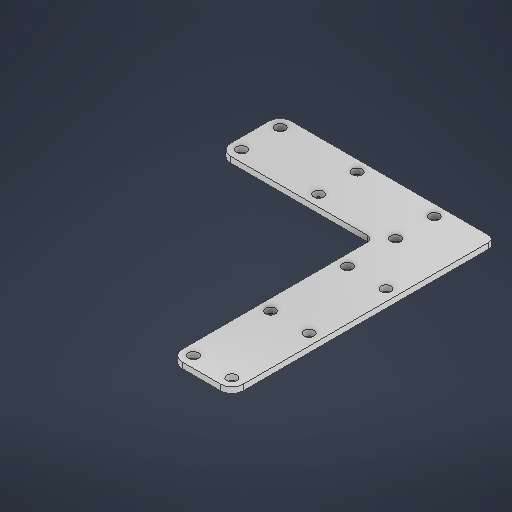
# Autodesk Inventor part: CNC-003-StructureGusset3
Saved by Autodesk Inventor 2026.2 (Build 302298000, 298)
## iProperties
Created: 2026-06-14
Part Number: CNC-003-StructureGusset3
Material: Steel AISI 1080
Document SubType Name: Modeling
Designer: Kenji
Density: 7.85 g/cm^3
Appearance: Aluminum - Dark
Author: Kenji
Autodesk Inventor part; units mm, degrees
ref_plane "YZ Plane" through (0, 0, 0) normal (1, 0, 0) x (0, 1, 0)
ref_plane "XZ Plane" through (0, 0, 0) normal (0, 1, 0) x (-1, 0, 0)
ref_plane "XY Plane" through (0, 0, 0) normal (0, 0, 1) x (1, 0, 0)
sketch "Sketch1" plane through (0, 0, 0) normal (0, 1, 0) x (-1, 0, 0)
  circle A0 centre (0, 0) radius 2.6
  line L0 (0, 0) -> (0, -2.6) construction
  line L1 (0, 0) -> (-2.6, 0) construction
  circle A1 centre (-20, 0) radius 2.6
  circle A2 centre (0, 40) radius 2.6
  circle A3 centre (-20, 40) radius 2.6
  circle A4 centre (0, 80) radius 2.6
  circle A5 centre (-20, 80) radius 2.6
  circle A6 centre (0, -25) radius 2.6
  line L2 (0, -25) -> (2.6, -25) construction
  line L3 (0, -25) -> (0, -27.6) construction
  circle A7 centre (40, -25) radius 2.6
  circle A8 centre (80, -25) radius 2.6
  circle A9 centre (0, -45) radius 2.6
  circle A10 centre (40, -45) radius 2.6
  circle A11 centre (80, -45) radius 2.6
  circle A12 centre (0, 80) radius 5.775 construction
  circle A13 centre (-20, 80) radius 5.775 construction
  circle A14 centre (80, -45) radius 5.775 construction
  circle A15 centre (80, -25) radius 5.775 construction
  line L4 (5.775, 80) -> (5.775, -16.05)
  line L5 (0, 85.775) -> (-20, 85.775)
  arc A16 (5.775, 80) -> (0, 85.775) centre (0, 80) ccw
  arc A17 (-20, 85.775) -> (-25.775, 80) centre (-20, 80) ccw
  line L6 (80, -19.225) -> (8.95, -19.225)
  line L7 (-25.775, 80) -> (-25.775, -47.6)
  line L8 (-22.6, -50.775) -> (80, -50.775)
  arc A18 (-25.775, -47.6) -> (-22.6, -50.775) centre (-22.6, -47.6) ccw
  arc A19 (5.775, -16.05) -> (8.95, -19.225) centre (8.95, -16.05) ccw
  line L9 (85.775, -25) -> (85.775, -45)
  arc A20 (80, -50.775) -> (85.775, -45) centre (80, -45) ccw
  arc A21 (85.775, -25) -> (80, -19.225) centre (80, -25) ccw
  point P0 (-20, -2.6)
  point P1 (-22.6, 0)
  point P2 (0, 37.4)
  point P3 (-2.6, 40)
  point P4 (-20, 37.4)
  point P5 (-22.6, 40)
  point P6 (0, 77.4)
  point P7 (-2.6, 80)
  point P8 (-20, 77.4)
  point P9 (-22.6, 80)
  point P10 (42.6, -25)
  point P11 (40, -27.6)
  point P12 (82.6, -25)
  point P13 (80, -27.6)
  point P14 (2.6, -45)
  point P15 (0, -47.6)
  point P16 (42.6, -45)
  point P17 (40, -47.6)
  point P18 (82.6, -45)
  point P19 (80, -47.6)
  point P20 (5.775, -19.225)
  dimension "d0" = 5.2
  dimension "d3" = 20
  dimension "d6" = 40
  dimension "d13" = 40
  dimension "d16" = 20
  dimension "d19" = 3.175
  dimension "d23" = 25
  dimension "d24" = 3.175
  constraints: 45 point on circle, 22 centre point, 20 end point, 14 tangent, 9 equal radius, 5 vertical, 4 coincident, 4 horizontal, 3 perpendicular, 2 point on line, 1 vertical alignment, 40 other
  measures "d0" diameter of A0
  measures "d3" distance of L0.start A1.centre
  measures "d6" distance of L0.start A2.centre
  measures "d13" distance of L2.start A7.centre
  measures "d16" distance of L2.start A9.centre
  measures "d19" radial gap between concentric circles of A12 A4
  measures "d23" distance of L2.start point (0, 0)
  measures "d24" radius of A18
extrude "Extrusion2" add sketch "Sketch1" along normal blind 3
body "Solid2"
